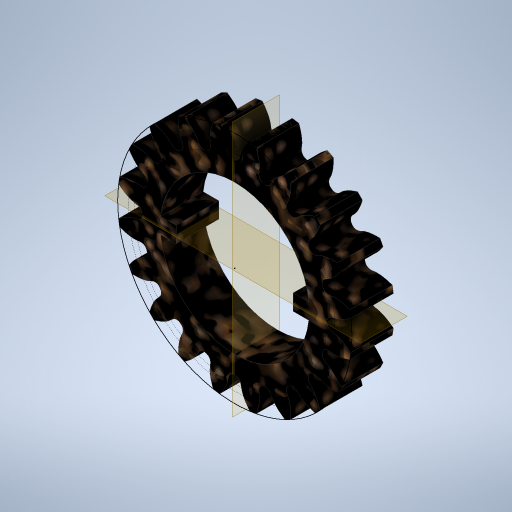
# Autodesk Inventor part: koloVelke
Saved by Autodesk Inventor 2023 (Build 270158000, 158)
## iProperties
Created: 2023-11-20
Part Number: koloVelke
Material: Generic
Document SubType Name: Modeling
Designer: alexa
Density: 1 g/cm^3
Appearance: Dirt - Dark Brown
Author: alexa
Autodesk Inventor part; units mm, degrees
ref_plane "XY Plane" through (0, 0, 0) normal (0, 0, 1) x (1, 0, 0)
sketch "Sketch1" plane through (0, 0, 0) normal (0, 0, 1) x (1, 0, 0)
  spline S0 degree 3 poles (-2.8116, 21.8196) (-2.7395, 21.7281) (-2.5954, 21.5452) (-2.3909, 21.2619) (-2.1955, 20.9723) (-2.0109, 20.6757) (-1.8381, 20.372) (-1.6786, 20.0611) (-1.5343, 19.7429) (-1.4077, 19.4171) (-1.3216, 19.1388) (-1.2667, 18.9123) (-1.2427, 18.7392) (-1.2235, 18.5657) (-1.192, 18.3937) (-1.1464, 18.225) (-1.0886, 18.0599) (-1.0129, 17.9021) (-0.9182, 17.7549) (-0.8036, 17.6224) (-0.6688, 17.5102) (-0.541, 17.4389) (-0.4324, 17.3967) (-0.348, 17.3738) (-0.262, 17.3581) (-0.1455, 17.3514) (0, 17.3554) (0.1455, 17.3514) (0.262, 17.3581) (0.348, 17.3738) (0.4324, 17.3967) (0.541, 17.4389) (0.6688, 17.5102) (0.8036, 17.6224) (0.9182, 17.7549) (1.0129, 17.9021) (1.0886, 18.0599) (1.1464, 18.225) (1.192, 18.3937) (1.2235, 18.5657) (1.2427, 18.7392) (1.2667, 18.9123) (1.3216, 19.1388) (1.4077, 19.4171) (1.5343, 19.7429) (1.6786, 20.0611) (1.8381, 20.372) (2.0109, 20.6757) (2.1955, 20.9723) (2.3909, 21.2619) (2.5954, 21.5452) (2.7395, 21.7281) (2.8116, 21.8196) knots 0 0 0 0 0.03493 0.069861 0.104791 0.139721 0.17465 0.20958 0.244508 0.279434 0.314357 0.33182 0.349278 0.36674 0.384205 0.401666 0.419128 0.436589 0.454045 0.471499 0.488944 0.506391 0.515125 0.523853 0.532587 0.541315 0.558781 0.576247 0.584975 0.593709 0.602437 0.611171 0.628618 0.646064 0.663517 0.680973 0.698434 0.715896 0.733357 0.750822 0.768284 0.785742 0.803205 0.838128 0.873054 0.907983 0.942912 0.977841 1.012771 1.047701 1.082632 1.117562 1.117562 1.117562 1.117562
  circle A0 centre (0, 0) radius 17.3538 construction
  circle A1 centre (0, 0) radius 18.7939 construction
  circle A2 centre (0, 0) radius 20 construction
  circle A3 centre (0, 0) radius 22
  point P0 (-2.5974, 21.5437)
  point P1 (-2.3924, 21.2608)
  point P2 (-2.1973, 20.9711)
  point P3 (-2.0129, 20.6745)
  point P4 (-1.8403, 20.3708)
  point P5 (-1.6811, 20.0599)
  point P6 (-1.5373, 19.7416)
  point P7 (-1.4116, 19.4157)
  point P8 (-1.309, 19.0819)
  point P9 (-1.2696, 18.9118)
  point P10 (-1.2435, 18.7392)
  point P11 (-1.2214, 18.5659)
  point P12 (-1.1897, 18.3942)
  point P13 (-1.1444, 18.2256)
  point P14 (-1.0856, 18.0611)
  point P15 (-1.0098, 17.9039)
  point P16 (-0.9149, 17.7573)
  point P17 (-0.8002, 17.6257)
  point P18 (-0.6657, 17.5146)
  point P19 (-0.5134, 17.4296)
  point P20 (-0.4319, 17.3982)
  point P21 (-0.3478, 17.375)
  point P22 (-0.2617, 17.3598)
  point P23 (-0.1747, 17.3539)
  point P24 (0, 17.3538)
  point P25 (0.1747, 17.3539)
  point P26 (0.2617, 17.3598)
  point P27 (0.3478, 17.375)
  point P28 (0.4319, 17.3982)
  point P29 (0.5134, 17.4296)
  point P30 (0.6657, 17.5146)
  point P31 (0.8002, 17.6257)
  point P32 (0.9149, 17.7573)
  point P33 (1.0098, 17.9039)
  point P34 (1.0856, 18.0611)
  point P35 (1.1444, 18.2256)
  point P36 (1.1897, 18.3942)
  point P37 (1.2214, 18.5659)
  point P38 (1.2435, 18.7392)
  point P39 (1.2696, 18.9118)
  point P40 (1.309, 19.0819)
  point P41 (1.4116, 19.4157)
  point P42 (1.5373, 19.7416)
  point P43 (1.6811, 20.0599)
  point P44 (1.8403, 20.3708)
  point P45 (2.0129, 20.6745)
  point P46 (2.1973, 20.9711)
  point P47 (2.3924, 21.2608)
  point P48 (2.5974, 21.5437)
  constraints: 4 centre point, 2 point on circle, 107 other
extrude "Extrusion1" add sketch "Sketch1" against normal blind 8
extrude "Extrusion2" cut sketch "Sketch1" against normal blind 10 contours A3 S0 picked at (0.3079, 20.2554)
pattern_circular "Circular Pattern1" count 20 over 360 about axis through (0, 0, -10) along (0, 0, 1) of "Extrusion2"
sketch "Sketch2" plane through (0, 0, 0) normal (0, 0, 1) x (1, 0, 0)
  circle A0 centre (0, 0) radius 14
  line L0 (-17, 1.5) -> (-11, 1.5)
  line L1 (-11, 1.5) -> (-11, -1.5)
  line L2 (-11, -1.5) -> (-17, -1.5)
  line L3 (-17, -1.5) -> (-17, 1.5)
  line L4 (-17, 1.5) -> (-11, -1.5) construction
  line L5 (-11, 1.5) -> (-17, -1.5) construction
  line L6 (17, 1.5) -> (11, 1.5)
  line L7 (11, 1.5) -> (11, -1.5)
  line L8 (11, -1.5) -> (17, -1.5)
  line L9 (17, -1.5) -> (17, 1.5)
  line L10 (17, 1.5) -> (11, -1.5) construction
  line L11 (11, 1.5) -> (17, -1.5) construction
  point P0 (-14, 0)
  point P1 (14, 0)
  point P2 (-13.9194, -1.5)
  point P3 (13.9194, -1.5)
  point P4 (13.9194, 1.5)
  point P5 (-13.9194, 1.5)
  dimension "d7" = 28
  dimension "d8" = 3
  dimension "d10" = 6
  constraints: 24 end point, 4 midpoint, 4 parallel, 2 equal length, 2 horizontal, 2 perpendicular, 2 point on circle, 1 centre point, 1 coincident, 1 point on line
  measures "d7" diameter of A0
  measures "d8" distance of L0.end L1.end
  measures "d10" distance of L0.start L0.end
extrude "Extrusion3" cut sketch "Sketch2" against normal blind 10 contours L6 L7 L8 A0 L2 L1 L0
equation "\"d0\" = FaceWidth"
equation "\"Module\" = 2"
equation "\"PressureAngle\" = 20deg"
equation "\"UnitProfileClearance\" = 0.25"
equation "\"UnitRoundRadius\" = 0.35"
equation "\"HeadDiameter\" = 44"
equation "\"RootDiameter\" = 34.70762"
equation "\"BaseDiameter\" = 37.5877"
equation "\"FaceWidth\" = 8"
equation "\"HelixAngle\" = 0"
equation "\"UnitCorrection\" = 0"
equation "\"UnitAddendumModification\" = 0"
equation "\"CircularPitch\" = 6.283185"
equation "\"UnitBacklashShift\" = -0.073095"
equation "\"TotalToolShift\" = -0.14619"
equation "\"IsInternal\" = 0"
body "Solid1"
